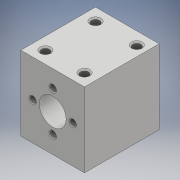
# Autodesk Inventor part: Z-AXIS SCREW SEAT
Saved by Autodesk Inventor 2018 (Build 220112000, 112)
## iProperties
Created: 2018-10-15
Part Number: Z-AXIS SCREW SEAT
Material: Generic
Document SubType Name: Modeling
Designer: Matthew Morey
Density: 1 g/cm^3
Appearance: Default
Author: Matthew Morey
Autodesk Inventor part; units mm, degrees
ref_plane "YZ Plane" through (0, 0, 0) normal (1, 0, 0) x (0, 1, 0)
ref_plane "XZ Plane" through (0, 0, 0) normal (0, 1, 0) x (-1, 0, 0)
ref_plane "XY Plane" through (0, 0, 0) normal (0, 0, 1) x (1, 0, 0)
sketch "Sketch1" plane through (0, 0, 0) normal (0, 1, 0) x (-1, 0, 0)
  line L0 (12.7, 14.875) -> (-12.7, 14.875)
  line L1 (-12.7, 14.875) -> (-12.7, -14.875)
  line L2 (-12.7, -14.875) -> (12.7, -14.875)
  line L3 (12.7, -14.875) -> (12.7, 14.875)
  point P0 (0, 0)
  dimension "d0" = 29.75
  dimension "d1" = 25.4
  dimension "d2" = 12.7
  dimension "d3" = 14.875
  constraints: 8 end point, 2 parallel, 1 horizontal, 1 perpendicular
  measures "d0" distance of L2.end L0.start
  measures "d1" distance of L1.end L2.end
  measures "d2" distance from line of point (0, 0) L3
  measures "d3" distance from line of point (0, 0) L2
extrude "Extrusion1" add sketch "Sketch1" along normal blind 29.8
sketch "Sketch2" plane through (0, 29.8, 0) normal (0, 1, 0) x (1, 0, 0)
  circle A0 centre (0, 0) radius 5.35
  line L0 (12.7, 14.875) -> (-12.7, 14.875) projected
  line L1 (-12.7, 14.875) -> (-12.7, -14.875) projected
  line L2 (-12.7, -14.875) -> (12.7, -14.875) projected
  dimension "d7" = 10.7
  dimension "d8" = 14.875
  dimension "d9" = 12.7
  dimension "d12" = 14.875
  constraints: 1 centre point
  measures "d7" diameter of A0
  measures "d8" distance from line of L0 A0.centre
  measures "d9" distance from line of L1 A0.centre
  measures "d12" distance from line of L2 A0.centre
extrude "Extrusion2" cut sketch "Sketch2" against normal through all
sketch "Sketch3" plane through (-12.7, 0, 14.875) normal (0, 0, 1) x (1, 0, 0)
  circle A0 centre (4.9, 24.9) radius 1.9
  circle A1 centre (21.4, 24.9) radius 1.9
  circle A2 centre (20.5, 4.9) radius 1.9
  circle A3 centre (4.9, 4.9) radius 1.9
  line L0 (0, 29.8) -> (25.4, 29.8) projected
  line L1 (0, 0) -> (0, 29.8) projected
  line L2 (0, 0) -> (25.4, 0) projected
  line L3 (25.4, 0) -> (25.4, 29.8) projected
  point P0 (12.7, 0)
  dimension "d13" = 3.8
  dimension "d14" = 3.8
  dimension "d15" = 3.8
  dimension "d16" = 3.8
  dimension "d17" = 4.9
  dimension "d18" = 4.9
  dimension "d19" = 4.9
  dimension "d20" = 4.9
  dimension "d21" = 4.9
  dimension "d22" = 4.9
  dimension "d23" = 4.9
  dimension "d24" = 4
  constraints: 4 centre point
  measures "d13" diameter of A0
  measures "d14" diameter of A1
  measures "d15" diameter of A2
  measures "d16" diameter of A3
  measures "d17" distance from line of L0 A0.centre
  measures "d18" distance from line of L1 A0.centre
  measures "d19" distance from line of L1 A3.centre
  measures "d20" distance from line of L2 A3.centre
  measures "d21" distance from line of L2 A2.centre
  measures "d22" distance from line of L3 A2.centre
  measures "d23" distance from line of L0 A1.centre
  measures "d24" distance from line of L3 A1.centre
hole "Hole1" at (-7.8, 24.9, 14.875) at (8.7, 24.9, 14.875) at (7.8, 4.9, 14.875) at (-7.8, 4.9, 14.875) direction (0, 0, -1) diameter 3.242 depth 11 tip angle 118 countersink diameter 4.3 countersink angle 90 thread size "M4x0.7" class "6H" standard "ANSI Metric M Profile"
sketch "Sketch4" plane through (0, 0, 0) normal (0, -1, 0) x (1, 0, 0)
  circle A0 centre (8, 0) radius 1.5
  circle A1 centre (0, -8) radius 1.5
  circle A2 centre (-8, 0) radius 1.5
  circle A3 centre (0, 8) radius 1.5
  line L0 (12.7, 14.875) -> (12.7, -14.875) projected
  line L1 (-12.7, -14.875) -> (-12.7, 14.875) projected
  line L2 (-12.7, 14.875) -> (12.7, 14.875) projected
  line L3 (12.7, -14.875) -> (-12.7, -14.875) projected
  point P0 (0, 0)
  dimension "d32" = 3
  dimension "d33" = 3
  dimension "d34" = 8
  dimension "d35" = 8
  dimension "d36" = 3
  dimension "d37" = 3
  dimension "d38" = 8
  dimension "d39" = 8
  dimension "d40" = 12.7
  dimension "d41" = 12.7
  dimension "d42" = 14.875
  dimension "d43" = 14.875
  constraints: 4 centre point
  measures "d32" diameter of A0
  measures "d33" diameter of A1
  measures "d34" distance of point (0, 0) A0.centre
  measures "d35" distance of point (0, 0) A1.centre
  measures "d36" diameter of A2
  measures "d37" diameter of A3
  measures "d38" distance of A2.centre point (0, 0)
  measures "d39" distance of A3.centre point (0, 0)
  measures "d40" distance from line of L0 A1.centre
  measures "d41" distance from line of A3.centre L1
  measures "d42" distance from line of L2 A0.centre
  measures "d43" distance from line of L3 A2.centre
hole "Hole2" at (8, 0, 0) at (0, 0, -8) at (-8, 0, 0) at (0, 0, 8) direction (0, 1, 0) diameter 2.459 depth 10 tip angle 118 countersink diameter 3.01 countersink angle 90 thread size "M3x0.5" class "6H" standard "ANSI Metric M Profile"
body "Solid1"
